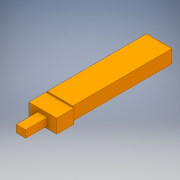
# Autodesk Inventor part: Battery_small
Saved by Autodesk Inventor 2018 (Build 220112000, 112)
## iProperties
Created: 2017-12-31
Part Number: Battery_small
Material: Generic
Document SubType Name: Modeling
Designer: suchanek
Density: 1 g/cm^3
Appearance: Default
Author: suchanek
Autodesk Inventor part; units mm, degrees
ref_plane "YZ Plane" through (0, 0, 0) normal (1, 0, 0) x (0, 1, 0)
ref_plane "XZ Plane" through (0, 0, 0) normal (0, 1, 0) x (-1, 0, 0)
ref_plane "XY Plane" through (0, 0, 0) normal (0, 0, 1) x (1, 0, 0)
sketch "Sketch2" plane through (0, 0, 0) normal (0, 1, 0) x (-1, 0, 0)
  line L0 (0, 0) -> (5.5, 0)
  line L1 (5.5, 0) -> (5.5, 3)
  line L2 (5.5, 3) -> (0, 3)
  line L3 (0, 3) -> (0, 0)
  line L4 (5.5, 3) -> (-6.7, 3)
  line L5 (-6.7, 3) -> (-6.7, -3.1)
  line L6 (-6.7, -3.1) -> (5.5, -3.1)
  line L7 (5.5, -3.1) -> (5.5, 3)
  dimension "d0" = 5.5
  dimension "d1" = 3
  dimension "d2" = 12.2
  dimension "d3" = 6.1
  constraints: 16 end point, 4 parallel, 2 horizontal, 2 perpendicular
  measures "d0" distance of L2.end L1.end
  measures "d1" distance of L1.end L0.end
  measures "d2" distance of L6.end L5.end
  measures "d3" distance of L5.end L4.end
extrude "Extrusion1" add sketch "Sketch2" along normal blind 7.5
sketch "Sketch3" plane through (0, 7.5, 0) normal (0, 1, 0) x (1, 0, 0)
  line L0 (6.2, 2.1) -> (-5, 2.1)
  line L1 (-5, 2.1) -> (-5, -3.6)
  line L2 (-5, -3.6) -> (6.2, -3.6)
  line L3 (6.2, -3.6) -> (6.2, 2.1)
  line L4 (6.7, 3.1) -> (-5.5, 3.1) projected
  line L5 (6.7, -3) -> (6.7, 3.1) projected
  point P0 (0, 0)
  dimension "d6" = 6.7
  dimension "d7" = 5.7
  dimension "d8" = 11.2
  dimension "d9" = 0.5
  constraints: 8 end point, 2 parallel, 1 horizontal, 1 perpendicular
  measures "d6" distance between parallel lines of L2 L4
  measures "d7" distance between parallel lines of L2 L0
  measures "d8" distance between parallel lines of L1 L3
  measures "d9" distance between parallel lines of L3 L5
extrude "Extrusion2" add sketch "Sketch3" along normal blind 43.5
sketch "Sketch4" plane through (0, 0, 0) normal (0, -1, 0) x (1, 0, 0)
  line L0 (-1.45, -1.9) -> (2.65, -1.9)
  line L1 (2.65, -1.9) -> (2.65, 1.3)
  line L2 (2.65, 1.3) -> (-1.45, 1.3)
  line L3 (-1.45, 1.3) -> (-1.45, -1.9)
  line L4 (-5.5, 3) -> (6.7, 3) projected
  line L5 (-5.5, -3.1) -> (-5.5, 3) projected
  point P0 (0, 0)
  dimension "d12" = 3.2
  dimension "d13" = 4.1
  dimension "d14" = 1.7
  dimension "d15" = 4.05
  constraints: 8 end point, 2 parallel, 1 horizontal, 1 perpendicular
  measures "d12" distance between parallel lines of L2 L0
  measures "d13" distance of L1.end L2.end
  measures "d14" distance between parallel lines of L4 L2
  measures "d15" distance between parallel lines of L5 L3
extrude "Extrusion3" add sketch "Sketch4" along normal blind 9.5
body "Solid1"
